4mm_closing tool (Autodesk Fusion 360 design; units mm, degrees)
Autodesk Fusion 360 part; units mm, degrees
note: some values were not read from the file. Set by a fixed rule: which sketch regions a step uses.
sketch "Sketch1" plane through (0, 0, 0) normal (0, 1, 0) x (1, 0, 0)
  line L0 (0, -0.5) -> (0, -10)
  line L1 (0, -10) -> (-22, -10)
  line L2 (-22, -10) -> (-22, -4.25)
  line L3 (-22, -4.25) -> (-20, -2.25)
  line L4 (-3, -2.25) -> (-3, -0.5)
  line L5 (-3, -0.5) -> (0, -0.5)
  line L6 (-20, -2.25) -> (-3, -2.35)
  line L7 (-3, -2.35) -> (-3, -2.25)
  dimension "d1" = 3
  dimension "d4" = 19
  dimension "d5" = 2
  dimension "d6" = 2
  dimension "d9" = 0.5
  dimension "d19" = 10
  dimension "d28" = 0.1
  dimension "d29" = 2.25
  constraint vertical L0
  constraint perpendicular L0 L1
  constraint perpendicular L1 L2
  constraint perpendicular L0 L5
  constraint coincident L0.start L5.end
  constraint coincident origin L0
  constraint horizontal L3.end L4.start
  constraint vertical L4.start L6.end
  constraint vertical L4
  measures "d1" distance of L4.end L0.start
  measures "d4" distance of L2.end L4
  measures "d5" horizontal distance of L2.end L3.end
  measures "d6" vertical distance of L2.end L3.end
  measures "d9" vertical distance of origin L0.start
  measures "d19" distance of origin L1
  measures "d28" vertical distance of L4.start L6.end
  measures "d29" vertical distance of origin L3.end
revolve "Revolve1" add sketch "Sketch1" angle 360 about axis through (1.75, 0, 0) along (1, 0, 0)
sketch "Sketch2" plane through (-22, 0, 0) normal (-1, 0, 0) x (0, -1, 0)
  circle A0 centre (0, 0) radius 10
  circle A1 centre (0, 0) radius 4.25
  line L0 (4.5299, -4.4251) -> (-4.5299, -4.3938) construction
  line L1 (-4.5299, -4.3938) -> (-4.5414, -7.7238) construction
  line L2 (-4.5414, -7.7238) -> (4.5184, -7.7551) construction
  line L3 (4.5184, -7.7551) -> (4.5299, -4.4251) construction
  dimension "d8" = 3
  text T0 "4mm" font "Arial" height 3 align centre top in box 9.0598 x 3.3299 at (4.5299, -4.4251) x (-0.999994, 0.003455) y (-0.003455, -0.999994) spacing 1
  constraint vertical A0.centre
sketch "Sketch3" plane through (0, 0, 0) normal (1, 0, 0) x (0, 1, 0)
  circle A0 centre (0, 0) radius 0.5
  circle A1 centre (0, 0) radius 10
  line L0 (7.1208, 6.1179) -> (-6.5015, 6.1179) construction
  line L1 (-6.5015, 6.1179) -> (-6.5015, -1.3422) construction
  line L2 (-6.5015, -1.3422) -> (7.1208, -1.3422) construction
  line L3 (7.1208, -1.3422) -> (7.1208, 6.1179) construction
  dimension "d10" = 3.5
  text T0 "4 mm" font "Arial" height 3.5 align centre middle in box 13.6223 x 7.4601 at (7.1208, 6.1179) x (-1, 0) y (0, -1) spacing 1
emboss "Emboss1" depth -0.2 profiles "Sketch3" section 1 text T0 onto face at (0, 0.4968, 6.7961)
emboss "Emboss2" depth -0.05 profiles "Sketch2" section 1 text T0 onto face at (-22, 0.4968, 8.0461)
sketch "Sketch4" plane through (0, 0, 0) normal (0, 1, 0) x (1, 0, 0)
  line L0 (-16.9639, 3.5615) -> (-4.9727, 3.4531) construction
  line L1 (-4.9727, 3.4531) -> (-5.0361, -3.5615) construction
  line L2 (-5.0361, -3.5615) -> (-17.0273, -3.4531) construction
  line L3 (-17.0273, -3.4531) -> (-16.9639, 3.5615) construction
  dimension "d20" = 3
  text T0 "4 mm" font "Arial" height 3 align centre top in box 11.9918 x 7.0149 at (-16.9639, 3.5615) x (0.999959, -0.009043) y (-0.009043, -0.999959) spacing 1 mirrored across
emboss "Emboss3" depth -0.4 profiles "Sketch4" section 1 text T0 onto face at (-14.6667, 0.9957, 9.9503)
pattern_circular "C-Pattern1" count 3 over 360 about axis through (1.75, 0, 0) along (1, 0, 0) of "Emboss3"
fillet "Fillet1" radius 0.5 2 edges at (-22, -3.6162, -9.3233) (0, -3.6162, -9.3233)
equation "d29 = ( 4.5 / 2 ) * 1 mm"
